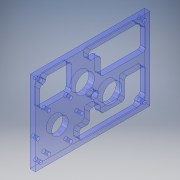
# Autodesk Inventor part: InsideMotorPlate
Saved by Autodesk Inventor 2019 (Build 230136000, 136)
## iProperties
Created: 2020-02-28
Part Number: InsideMotorPlate
Material: Aluminum 6061
Document SubType Name: Modeling
Designer: james
Density: 2.7 g/cm^3
Appearance: Clear - Blue
Mass: 134.969 g
Surface Area: 248.661 cm^2
Volume: 49.9883 cm^3
Author: james
Autodesk Inventor part; units mm, degrees
ref_plane "YZ Plane" through (0, 0, 0) normal (1, 0, 0) x (0, 1, 0)
ref_plane "XZ Plane" through (0, 0, 0) normal (0, 1, 0) x (-1, 0, 0)
ref_plane "XY Plane" through (0, 0, 0) normal (0, 0, 1) x (1, 0, 0)
sketch "Sketch1" plane through (0, 0, 0) normal (1, 0, 0) x (0, 1, 0)
  line L0 (46.7204, 78.4349) -> (-48.5296, 78.4349)
  line L1 (-48.5296, 78.4349) -> (-48.5296, -54.9151)
  line L2 (-48.5296, -54.9151) -> (46.7204, -54.9151)
  line L3 (46.7204, -54.9151) -> (46.7204, 78.4349)
  point P0 (0, 0)
  dimension "d0" = 133.35
  dimension "d1" = 95.25
  constraints: 8 end point, 2 parallel, 1 horizontal, 1 perpendicular
  measures "d0" distance of L2.end L0.start
  measures "d1" distance of L0.start L0.end
extrude "Extrusion1" add sketch "Sketch1" along normal blind 6.35
sketch "Sketch2" plane through (6.35, 0, 0) normal (1, 0, 0) x (0, 0, -1)
  line L0 (54.9151, 46.7204) -> (-78.4349, 46.7204) projected
  line L1 (-78.4349, 46.7204) -> (-78.4349, -48.5296) projected
  line L2 (-78.4349, -48.5296) -> (54.9151, -48.5296) projected
  line L3 (54.9151, -48.5296) -> (54.9151, 46.7204) projected
  point P0 (0, 0)
  point P1 (-72.0849, 40.3704)
  point P2 (48.5651, 40.3704)
  point P3 (48.5651, -42.1796)
  point P4 (-72.0849, -42.1796)
  dimension "d4" = 0
  dimension "d5" = 0
  dimension "d6" = 0
  dimension "d7" = 0
  dimension "d8" = 6.35
  dimension "d9" = 6.35
  dimension "d10" = 6.35
  dimension "d11" = 6.35
  measures "d4" horizontal distance of point (-72.085, -42.18) point (-72.085, 40.37)
  measures "d5" horizontal distance of point (48.565, 40.37) point (48.565, -42.18)
  measures "d6" vertical distance of point (-72.085, -42.18) point (48.565, -42.18)
  measures "d7" vertical distance of point (-72.085, 40.37) point (48.565, 40.37)
  measures "d8" distance from line of L0 point (-72.085, 40.37)
  measures "d9" distance from line of L1 point (-72.085, 40.37)
  measures "d10" distance from line of L2 point (-72.085, -42.18)
  measures "d11" distance from line of L3 point (48.565, -42.18)
hole "Hole1" at (6.35, 40.3704, 72.0849) at (6.35, 40.3704, -48.5651) at (6.35, -42.1796, -48.5651) at (6.35, -42.1796, 72.0849) direction (-1, 0, 0) diameter 4.318 end through all
sketch "Sketch3" plane through (6.35, 0, 0) normal (1, 0, 0) x (0, 0, -1)
  circle A0 centre (-49.8599, -16.7796) radius 9.652
  line L0 (-78.4349, -48.5296) -> (54.9151, -48.5296) projected
  line L1 (-78.4349, 46.7204) -> (-78.4349, -48.5296) projected
  point P0 (0, 0)
  dimension "d19" = 19.304
  dimension "d20" = 31.75
  dimension "d21" = 28.575
  constraints: 1 centre point
  measures "d19" diameter of A0
  measures "d20" distance from line of L0 A0.centre
  measures "d21" distance from line of L1 A0.centre
extrude "Extrusion2" cut sketch "Sketch3" against normal blind 61.9125
sketch "Sketch4" plane through (6.35, 0, 0) normal (1, 0, 0) x (0, 0, -1)
  circle A0 centre (-49.8599, -16.7796) radius 9.652 projected
  circle A1 centre (-49.8599, -16.7796) radius 9.652 projected
  circle A2 centre (-49.8599, -16.7796) radius 25.4
  line L0 (-49.8599, -16.7796) -> (-108.2264, -16.7796)
  line L1 (-49.8599, -16.7796) -> (-68.0839, 14.7853)
  line L2 (-49.8599, -16.7796) -> (-30.0658, 17.5048)
  line L3 (-49.8599, -16.7796) -> (-1.4138, -16.7796)
  line L4 (-49.8599, -16.7796) -> (-32.2617, -47.2605)
  line L5 (-49.8599, -16.7796) -> (-70.9793, -53.3594)
  point P0 (0, 0)
  point P1 (-75.2599, -16.7796)
  point P2 (-24.4599, -16.7796)
  point P3 (-62.5599, 5.2174)
  point P4 (-37.1599, 5.2174)
  point P5 (-37.1599, -38.7767)
  point P6 (-62.5599, -38.7767)
  dimension "d24" = 50.8
  dimension "d25" = 60
  dimension "d26" = 60
  dimension "d27" = 60
  dimension "d28" = 60
  constraints: 12 end point, 6 point on circle, 5 point on line, 2 horizontal, 1 centre point, 1 coincident
  measures "d24" diameter of A2
  measures "d25" angle of L0 L1
  measures "d26" angle of L1 L2
  measures "d27" angle of L4 L3
  measures "d28" angle of L5 L0
hole "Hole2" at (6.35, -16.7796, 75.2599) at (6.35, -16.7796, 24.4599) at (6.35, 5.2174, 62.5599) at (6.35, 5.2174, 37.1599) at (6.35, -38.7767, 37.1599) at (6.35, -38.7767, 62.5599) direction (-1, 0, 0) diameter 4.318 end through all
sketch "Sketch5" plane through (6.35, 0, 0) normal (1, 0, 0) x (0, 0, -1)
  circle A0 centre (-20.9622, 11.7954) radius 11.1125
  circle A1 centre (-49.8599, -16.7796) radius 9.652 projected
  circle A2 centre (-49.8599, -16.7796) radius 40.64
  point P0 (0, 0)
  dimension "d37" = 81.28
  dimension "d36" = 22.225
  dimension "d44" = 28.575
  constraints: 1 centre point, 1 coincident, 3 other
  measures "d36" diameter of A0
  measures "d44" vertical distance of A1.centre A0.centre
extrude "Extrusion3" cut sketch "Sketch5" against normal blind 66.675 contours A0 A2 | A2 A0 picked at (-18.3231, 14.2307) picked at (-23.6766, 9.1113)
sketch "Sketch6" plane through (6.35, 0, 0) normal (1, 0, 0) x (0, 0, -1)
  circle A0 centre (-20.9622, 11.7954) radius 11.1125 projected
  circle A1 centre (-20.9622, 11.7954) radius 40.64
  circle A2 centre (10.7624, -13.6046) radius 11.1125
  point P0 (0, 0)
  dimension "d43" = 81.28
  dimension "d40" = 22.225
  dimension "d45" = 25.4
  constraints: 1 centre point, 1 coincident, 3 other
  measures "d40" diameter of A2
  measures "d45" vertical distance of A2.centre A0.centre
extrude "Extrusion4" cut sketch "Sketch6" against normal blind 39.6875 contours A2 A1 | A1 A2 picked at (7.7825, -11.2188) picked at (13.4712, -15.9622)
sketch "Sketch9" plane through (6.35, 0, 0) normal (1, 0, 0) x (0, 0, -1)
  line L0 (-63.6501, 41.6404) -> (-39.6177, 41.6404)
  line L1 (-36.4427, 38.4654) -> (-36.4427, 14.0798)
  line L2 (-2.8893, 28.3994) -> (-2.8893, 12.3805)
  line L3 (0.2857, 9.2055) -> (46.6601, 9.2055)
  line L4 (49.8351, 12.3805) -> (49.8351, 32.1154)
  line L5 (-12.39, -16.6835) -> (-6.0643, -16.6835)
  line L6 (-2.8893, -19.8585) -> (-2.8893, -25.1589)
  line L7 (-15.565, -28.2347) -> (-15.565, -19.8585)
  line L8 (46.6601, -5.3126) -> (28.4332, -5.3126)
  line L9 (25.2582, -8.4876) -> (25.2582, -25.1589)
  line L10 (46.6601, -37.0996) -> (46.6601, -37.0996)
  line L11 (49.8351, -33.9246) -> (49.8351, -8.4876)
  line L12 (22.0832, -28.3339) -> (0.2857, -28.3339)
  line L13 (-6.4311, -43.4496) -> (40.3101, -43.4496)
  line L14 (43.4851, -40.2746) -> (43.4851, -40.2746)
  line L15 (-18.74, -31.4097) -> (-24.3201, -31.4097)
  line L16 (-27.4951, -34.5847) -> (-27.4951, -40.2746)
  line L17 (-24.3201, -43.4496) -> (-6.4311, -43.4496)
  line L18 (40.3101, 41.6404) -> (-13.5085, 41.6404)
  line L19 (-16.6835, 38.4654) -> (-16.6835, 34.7494)
  line L20 (-13.5085, 31.5744) -> (-6.0643, 31.5744)
  line L21 (-66.8149, 38.211) -> (-66.8558, 38.7198)
  line L22 (-63.1337, 10.9048) -> (-39.6177, 10.9048)
  line L23 (-10.3395, -2.3301) -> (-7.9284, -2.3301)
  line L24 (-4.7534, -5.5051) -> (-4.7534, -6.425)
  line L25 (-7.9284, -9.6) -> (-10.3395, -9.6)
  line L26 (-13.5145, -6.425) -> (-13.5145, -5.5051)
  arc A0 (-10.3395, -2.3301) -> (-13.5145, -5.5051) centre (-10.3395, -5.5051) ccw
  arc A1 (-13.5145, -6.425) -> (-10.3395, -9.6) centre (-10.3395, -6.425) ccw
  arc A2 (-7.9284, -9.6) -> (-4.7534, -6.425) centre (-7.9284, -6.425) ccw
  arc A3 (-4.7534, -5.5051) -> (-7.9284, -2.3301) centre (-7.9284, -5.5051) ccw
  arc A4 (-18.74, -31.4097) -> (-15.565, -28.2347) centre (-18.74, -28.2347) ccw
  arc A5 (-24.3201, -31.4097) -> (-27.4951, -34.5847) centre (-24.3201, -34.5847) ccw
  arc A6 (-27.4951, -40.2746) -> (-24.3201, -43.4496) centre (-24.3201, -40.2746) ccw
  arc A7 (-12.39, -16.6835) -> (-15.565, -19.8585) centre (-12.39, -19.8585) ccw
  arc A8 (-2.8893, -19.8585) -> (-6.0643, -16.6835) centre (-6.0643, -19.8585) ccw
  arc A9 (-2.8893, -25.1589) -> (0.2857, -28.3339) centre (0.2857, -25.1589) ccw
  arc A10 (-63.6501, 41.6404) -> (-66.8149, 38.211) centre (-63.6501, 38.4654) ccw
  arc A11 (-39.6177, 10.9048) -> (-36.4427, 14.0798) centre (-39.6177, 14.0798) ccw
  arc A12 (-36.4427, 38.4654) -> (-39.6177, 41.6404) centre (-39.6177, 38.4654) ccw
  arc A13 (-2.8893, 28.3994) -> (-6.0643, 31.5744) centre (-6.0643, 28.3994) ccw
  arc A14 (-16.6835, 34.7494) -> (-13.5085, 31.5744) centre (-13.5085, 34.7494) ccw
  arc A15 (-13.5085, 41.6404) -> (-16.6835, 38.4654) centre (-13.5085, 38.4654) ccw
  arc A16 (46.6601, 9.2055) -> (49.8351, 12.3805) centre (46.6601, 12.3805) ccw
  arc A17 (-2.8893, 12.3805) -> (0.2857, 9.2055) centre (0.2857, 12.3805) ccw
  arc A18 (46.6601, -37.0996) -> (43.4851, -40.2746) centre (46.6601, -40.2746) ccw
  arc A19 (46.6601, -37.0996) -> (49.8351, -33.9246) centre (46.6601, -33.9246) ccw
  arc A20 (49.8351, -8.4876) -> (46.6601, -5.3126) centre (46.6601, -8.4876) ccw
  arc A21 (28.4332, -5.3126) -> (25.2582, -8.4876) centre (28.4332, -8.4876) ccw
  arc A22 (22.0832, -28.3339) -> (25.2582, -25.1589) centre (22.0832, -25.1589) ccw
  arc A23 (40.3101, -43.4496) -> (43.4851, -40.2746) centre (40.3101, -40.2746) ccw
  line L27 (-54.5967, 10.9048) -> (-70.1799, 10.9048)
  line L28 (-73.3549, 14.0798) -> (-73.3549, 32.1154)
  line L29 (-70.1799, 35.2904) -> (-70.0206, 35.2904)
  line L30 (-54.5967, 32.5043) -> (-54.5967, 31.5744)
  arc A24 (-70.0206, 35.2904) -> (-66.8558, 38.7198) centre (-70.0206, 38.4654) ccw
  arc A25 (-70.1799, 35.2904) -> (-73.3549, 32.1154) centre (-70.1799, 32.1154) ccw
  arc A26 (-73.3549, 14.0798) -> (-70.1799, 10.9048) centre (-70.1799, 14.0798) ccw
  line L31 (54.9151, 46.7204) -> (-78.4349, 46.7204) projected
  line L32 (-78.4349, 46.7204) -> (-78.4349, -48.5296) projected
  line L33 (54.9151, -48.5296) -> (54.9151, 46.7204) projected
  line L34 (-78.4349, -48.5296) -> (54.9151, -48.5296) projected
  line L35 (43.4851, 38.4654) -> (43.4851, 38.4654)
  line L36 (46.6601, 35.2904) -> (46.6601, 35.2904)
  circle A27 centre (48.5651, 40.3704) radius 2.159 projected
  arc A28 (43.4851, 38.4654) -> (40.3101, 41.6404) centre (40.3101, 38.4654) ccw
  arc A29 (43.4851, 38.4654) -> (46.6601, 35.2904) centre (46.6601, 38.4654) ccw
  arc A30 (49.8351, 32.1154) -> (46.6601, 35.2904) centre (46.6601, 32.1154) ccw
  circle A31 centre (-72.0849, 40.3704) radius 2.159 projected
  circle A32 centre (48.5651, -42.1796) radius 2.159 projected
  point P0 (0, 0)
  point P1 (43.4851, -43.4496)
  point P2 (-27.4951, -43.4496)
  point P3 (-13.5145, -2.3301)
  dimension "d56" = 3.175
  dimension "d57" = 3.175
  dimension "d58" = 3.175
  dimension "d61" = 3.175
  dimension "d62" = 3.175
  dimension "d63" = 5.08
  dimension "d64" = 5.08
  dimension "d65" = 5.08
  dimension "d66" = 5.08
  dimension "d67" = 5.08
  dimension "d68" = 5.08
  dimension "d69" = 5.08
  dimension "d70" = 5.08
  dimension "d71" = 3.175
  dimension "d72" = 5.08
  dimension "d73" = 5.08
  dimension "d74" = 5.08
  dimension "d75" = 5.08
  constraints: 66 end point, 60 point on circle, 60 tangent, 30 centre point, 24 equal radius, 11 parallel, 9 perpendicular, 9 point on line, 8 horizontal
  measures "d56" radius of A0
  measures "d57" radius of A10
  measures "d58" radius of A14
  measures "d61" radius of A23
  measures "d62" radius of A24
  measures "d63" distance between parallel lines of L31 L0
  measures "d64" distance between parallel lines of L32 L28
  measures "d65" distance between parallel lines of L31 L18
  measures "d66" distance between parallel lines of L33 L11
  measures "d67" distance between parallel lines of L34 L13
  measures "d68" distance between parallel lines of L33 L4
  measures "d69" distance from line of L35 A27.centre
  measures "d70" distance from line of L36 A27.centre
  measures "d71" radius of A28
  measures "d72" distance from line of A31.centre L21
  measures "d73" vertical distance of L29.end A31.centre
  measures "d74" horizontal distance of A32.centre L14.start
  measures "d75" vertical distance of A32.centre L10.end
extrude "Extrusion7" cut sketch "Sketch9" against normal blind 6.35 contours L0 A12 L1 A11 L22 L27 A26 L28 A25 L29 A24 L21 A10 | A13 L20 A14 L19 A15 L18 A28 A29 A30 L4 A16 L3 A17 L2 | L5 A8 L6 A9 L12 A22 L9 A21 L8 A20 L11 A19 A18 A23 L13 L17 A6 L16 A5 L15 A4 L7 A7 | L23 A3 L24 A2 L25 A1 L26 A0
body "Solid1"
